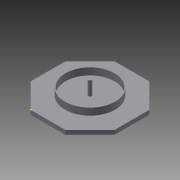
# Autodesk Inventor part: base
Saved by Autodesk Inventor 2015 (Build 190159000, 159)
## iProperties
Created: 2020-01-21
Part Number: base
Material: Generic
Document SubType Name: Modeling
Designer: hp
Density: 1 g/cm^3
Appearance: Default
Author: hp
Autodesk Inventor part; units mm, degrees
ref_plane "YZ Plane" through (0, 0, 0) normal (1, 0, 0) x (0, 1, 0)
ref_plane "XZ Plane" through (0, 0, 0) normal (0, 1, 0) x (-1, 0, 0)
ref_plane "XY Plane" through (0, 0, 0) normal (0, 0, 1) x (1, 0, 0)
sketch "Sketch1" plane through (0, 0, 0) normal (0, 1, 0) x (-1, 0, 0)
  line L0 (0, 19.6176) -> (898.0256, -878.408)
  line L1 (0, 19.6176) -> (1270, 19.6176) construction
  line L2 (0, 19.6176) -> (-1270, 19.6176)
  line L3 (-1270, 19.6176) -> (-2168.0256, -878.408)
  line L4 (-1270, 19.6176) -> (0, 19.6176) construction
  line L5 (898.0256, -878.408) -> (-2168.0256, -878.408)
  line L6 (898.0256, -878.408) -> (-2168.0256, -878.408)
  line L7 (-2168.0256, -878.408) -> (-2168.0256, -2148.408)
  line L8 (-2168.0256, -2148.408) -> (898.0256, -2148.408)
  line L9 (898.0256, -2148.408) -> (898.0256, -878.408)
  line L10 (898.0256, -2148.408) -> (0, -3046.4336)
  line L11 (898.0256, -2148.408) -> (2168.0256, -2148.408) construction
  line L12 (-2168.0256, -2148.408) -> (-1270, -3046.4336)
  line L13 (-1270, -3046.4336) -> (0, -3046.4336)
  point P0 (0, 0)
  dimension "d0" = 1270
  dimension "d1" = 45
  dimension "d2" = 1270
  dimension "d3" = 1270
  dimension "d4" = 135
  dimension "d5" = 1270
  dimension "d6" = 1270
  dimension "d7" = 135
  dimension "d8" = 1270
  constraints: 28 end point, 6 horizontal, 3 equal length, 2 parallel, 1 perpendicular
  measures "d0" distance of L0.start L0.end
  measures "d1" angle of L0 L1
  measures "d2" distance of L0.start L2.end
  measures "d3" distance of L2.end L3.end
  measures "d4" angle of L3 L4
  measures "d5" distance of L7.end L6.end
  measures "d6" distance of L8.end L10.end
  measures "d7" angle of L10 L11
  measures "d8" distance of L7.end L12.end
extrude "Extrusion1" add sketch "Sketch1" along normal blind 152.4
sketch "Sketch2" plane through (0, 152.4, 0) normal (0, 1, 0) x (1, 0, 0)
  circle A0 centre (623.2771, 1525.4657) radius 60.1528
  line L0 (2150.1664, 894.5684) -> (-903.6123, 2156.3631)
  line L1 (-903.6123, 2156.3631) -> (2150.1664, 2156.3631)
  line L2 (2150.1664, 2156.3631) -> (-903.6123, 894.5684)
  point P0 (0, 0)
  constraints: 6 end point, 2 midpoint, 1 centre point, 1 horizontal
extrude "Extrusion2" add sketch "Sketch2" along normal blind 508 contours A0 L0 L2 | L2 L0 A0 | A0 L2 L0 | L0 L2 A0
sketch "Sketch3" plane through (0, 152.4, 0) normal (0, 1, 0) x (1, 0, 0)
  point P0 (0, 0)
sketch "Sketch4" plane through (0, 152.4, 0) normal (0, 1, 0) x (1, 0, 0)
  line L0 (2168.5073, 886.5825) -> (-936.3093, 2164.3771)
  line L1 (-936.3093, 2164.3771) -> (2152.0565, 2164.3771)
  line L2 (2168.0256, 2148.408) -> (1270, 3046.4336) projected
  line L3 (2168.0256, 2148.408) -> (-889.8511, 886.5825)
  circle A0 centre (623.2771, 1525.4657) radius 60.1528 projected
  circle A1 centre (623.2771, 1525.4657) radius 914.8505
  circle A2 centre (623.2771, 1525.4657) radius 889.9971
  point P0 (0, 0)
  constraints: 6 end point, 2 centre point, 2 coincident, 1 horizontal, 1 point on line
extrude "Extrusion3" add sketch "Sketch4" along normal blind 254 contours A1 L3 A2 L0 | L0 A2 L3 A1 | A1 L0 A2 L3 | A1 L1 A2 L0 | L3 A2 L1 A1 | A1 L1 A2
body "Solid1"
